Autodesk Fusion 360 part; units mm, degrees
(part 2 of 2)
sketch "Sketch30" plane through (0, 0, 0) normal (0, -1, 0) x (1, 0, 0)
  line L0 (40, 0) -> (71.5, 0)
  line L1 (71.5, 0) -> (71.5, 10)
  line L2 (71.5, 10) -> (40, 10)
  line L3 (40, 10) -> (40, 0)
  line L4 (40, 10) -> (42, 10)
  line L5 (42, 10) -> (40, 0)
  line L6 (40, 0) -> (40, 10)
  line L7 (71.5, 10) -> (69.5, 10)
  line L8 (69.5, 10) -> (71.5, 0)
  line L9 (71.5, 0) -> (71.5, 10)
  dimension "d261" = 2
  constraint coincident L2.end L3.start
  constraint coincident L2 L4.end
  constraint coincident L0.start L3.end
  constraint coincident L1.end L2.start
  constraint perpendicular L1 L7
  constraint coincident L0.end L1.start
  measures "d261" distance of L1.end L7.end
sketch "Sketch31" plane through (71.5, 0, 0) normal (1, 0, 0) x (0, 0, -1)
  line L0 (0, 0) -> (0, 18)
  line L1 (0, 18) -> (-10, 18)
  line L2 (-10, 18) -> (-10, 0)
  line L3 (-10, 0) -> (0, 0)
  line L4 (-10, 0) -> (-10, 2)
  line L5 (-10, 2) -> (0, 0)
  line L6 (0, 0) -> (-10, 0)
  line L7 (-10, 18) -> (-10, 16)
  line L8 (-10, 16) -> (0, 18)
  line L9 (0, 18) -> (-10, 18)
  constraint coincident L2.end L3.start
  constraint coincident L2 L4.end
  constraint coincident L0.start L3.end
  constraint coincident L1.end L2.start
  constraint coincident L2 L7.end
  constraint coincident L0.end L1.start
extrude "Extrude32" cut sketch "Sketch31" against normal blind 40 contours L2 L3 L4 L5 L6 | L1 L2 L7 L8 L9 bodies 8
extrude "Extrude33" cut sketch "Sketch30" against normal blind 27 contours L2 L3 L4 L5 L6 | L1 L2 L7 L8 L9 bodies 8
shell "Shell9" thickness 1 removed faces 1 at (50.5, 12, 0) on bodies 8
sketch "Sketch32" plane through (0, 0, 9) normal (0, 0, -1) x (-1, 0, 0)
  line L0 (-68.6802, 15.1802) -> (-68.6802, 2.8198)
  line L1 (-68.6802, 2.8198) -> (-42.8198, 2.8198)
  line L2 (-42.8198, 2.8198) -> (-42.8198, 15.1802)
  line L3 (-42.8198, 15.1802) -> (-68.6802, 15.1802)
  line L4 (-56.3, 7) -> (-55.2, 7)
  line L5 (-55.2, 7) -> (-55.2, 11)
  line L6 (-55.2, 11) -> (-56.3, 11)
  line L7 (-56.3, 11) -> (-56.3, 7)
  line L8 (-53.75, 8.375) -> (-57.75, 8.375)
  line L9 (-57.75, 8.375) -> (-57.75, 9.625)
  line L10 (-57.75, 9.625) -> (-53.75, 9.625)
  line L11 (-53.75, 9.625) -> (-53.75, 8.375)
  line L12 (-57.3, 6) -> (-54.2, 6)
  line L13 (-54.2, 6) -> (-54.2, 12)
  line L14 (-54.2, 12) -> (-57.3, 12)
  line L15 (-57.3, 12) -> (-57.3, 6)
  line L16 (-58.75, 10.625) -> (-52.75, 10.625)
  line L17 (-52.75, 10.625) -> (-52.75, 7.375)
  line L18 (-52.75, 7.375) -> (-58.75, 7.375)
  line L19 (-58.75, 7.375) -> (-58.75, 10.625)
  dimension "d275" = 3.1
  dimension "d276" = 6
  dimension "d279" = 6
  dimension "d280" = 3.25
  constraint horizontal L4
  constraint vertical L5
  constraint horizontal L6
  constraint vertical L7
  constraint horizontal L8
  constraint vertical L9
  constraint horizontal L10
  constraint vertical L11
  constraint horizontal L12
  constraint vertical L13
  constraint horizontal L14
  constraint vertical L15
  constraint horizontal L16
  constraint vertical L17
  constraint horizontal L18
  constraint vertical L19
  measures "d275" distance of L12.start L12.end
  measures "d276" distance of L12.start L14.end
  measures "d279" distance of L16.start L16.end
  measures "d280" distance of L16.start L18.end
extrude "Extrude34" add sketch "Sketch32" along normal blind 9 contours L4 L5 L7 L12 L13 L15 L18 | L7 L8 L15 L18 | L5 L8 L13 L18 | L8 L9 L10 L15 L16 L18 L19 | L8 L10 L11 L13 L16 L17 L18 | L7 L10 L15 L16 | L5 L10 L13 L16 | L5 L6 L7 L13 L14 L15 L16 bodies 8
fillet "Fillet9" radius 1 8 edges at (55.75, 16, 10) (41, 17, 5) (42, 9, 10) (41, 1, 5) (55.75, 2, 10) (70.5, 17, 5) (69.5, 9, 10) (70.5, 1, 5) on bodies 8
move_body "Move13" bodies 8 to x (1, 0, 0) y (0, 1, 0) z (0, 0, 1) at (-55.7506, -8.335, 12.2427)
move_body "Move14" bodies 1 to x (1, 0, 0) y (0, 1, 0) z (0, 0, 1) at (70, 0, 0)
move_body "Move15" bodies 2 to x (1, 0, 0) y (0, 1, 0) z (0, 0, 1) at (-80, 0, 0)
move_body "Move16" bodies 3 to x (1, 0, 0) y (0, 1, 0) z (0, 0, 1) at (100, 0, 0)
move_body "Move17" bodies 4 to x (1, 0, 0) y (0, 1, 0) z (0, 0, 1) at (140, 0, 0)
move_body "Move18" bodies 5 to x (1, 0, 0) y (0, 1, 0) z (0, 0, 1) at (180, 0, 0)
move_body "Move19" bodies 6 to x (1, 0, 0) y (0, 1, 0) z (0, 0, 1) at (220, 0, 0)
move_body "Move20" bodies 7 to x (1, 0, 0) y (0, 1, 0) z (0, 0, 1) at (270, 0, 0)
move_body "Move21" bodies 8 to x (1, 0, 0) y (0, 1, 0) z (0, 0, 1) at (40, 0, 0)
move_body "Move22" bodies 2 to x (1, 0, 0) y (0, 1, 0) z (0, 0, 1) at (40, 0, 0)
sketch "Sketch33" plane through (0, 0, 0) normal (0, 0, 1) x (1, 0, 0)
  line L0 (-280, 0) -> (-167.5, 0)
  line L1 (-167.5, 0) -> (-167.5, 18)
  line L2 (-167.5, 18) -> (-280, 18)
  line L3 (-280, 18) -> (-280, 0)
  dimension "d285" = 112.5
  dimension "d286" = 18
  constraint horizontal L0
  constraint vertical L1
  constraint horizontal L2
  constraint vertical L3
  measures "d285" distance of L0.start L0.end
  measures "d286" distance of L0.start L2.end
extrude "Extrude35" add sketch "Sketch33" along normal blind 10 separate body makes body 9
sketch "Sketch34" plane through (0, 0, 0) normal (0, -1, 0) x (1, 0, 0)
  line L0 (-280, 0) -> (-167.5, 0)
  line L1 (-167.5, 0) -> (-167.5, 10)
  line L2 (-167.5, 10) -> (-280, 10)
  line L3 (-280, 10) -> (-280, 0)
  line L4 (-167.5, 10) -> (-169.5, 10)
  line L5 (-169.5, 10) -> (-167.5, 0)
  line L6 (-167.5, 0) -> (-167.5, 10)
  line L7 (-280, 10) -> (-278, 10)
  line L8 (-278, 10) -> (-280, 0)
  line L9 (-280, 0) -> (-280, 10)
  dimension "d289" = 2
  dimension "d290" = 2
  constraint coincident L1.end L2.start
  constraint perpendicular L1 L4
  constraint coincident L0.end L1.start
  constraint coincident L2.end L3.start
  constraint perpendicular L3 L7
  constraint coincident L0.start L3.end
  measures "d289" distance of L1.end L4.end
  measures "d290" distance of L2.end L7.end
sketch "Sketch35" plane through (-280, 0, 0) normal (-1, 0, 0) x (0, 0, 1)
  line L0 (0, 18) -> (0, 0)
  line L1 (0, 0) -> (10, 0)
  line L2 (10, 0) -> (10, 18)
  line L3 (10, 18) -> (0, 18)
  line L4 (10, 18) -> (10, 16)
  line L5 (10, 16) -> (0, 18)
  line L6 (0, 18) -> (10, 18)
  line L7 (10, 0) -> (10, 2)
  line L8 (10, 2) -> (0, 0)
  line L9 (0, 0) -> (10, 0)
  dimension "d291" = 2
  dimension "d292" = 2
  constraint coincident L2.end L3.start
  constraint perpendicular L3 L4
  constraint coincident L0.start L3.end
  constraint coincident L1.end L2.start
  constraint perpendicular L1 L7
  constraint coincident L0.end L1.start
  measures "d291" distance of L2.end L4.end
  measures "d292" distance of L1.end L7.end
extrude "Extrude36" cut sketch "Sketch35" against normal blind 120 contours L2 L3 L4 L5 L6 | L1 L2 L7 L8 L9 bodies 9
extrude "Extrude37" cut sketch "Sketch34" against normal blind 35 contours L2 L3 L7 L8 L9 | L1 L2 L4 L5 L6 bodies 9
shell "Shell10" thickness 1 removed faces 1 at (-242.5, 6, 0) on bodies 9
sketch "Sketch36" plane through (0, 0, 9) normal (0, 0, -1) x (-1, 0, 0)
  line L0 (277.1802, 2.8198) -> (277.1802, 15.1802)
  line L1 (277.1802, 15.1802) -> (170.3198, 15.1802)
  line L2 (170.3198, 15.1802) -> (170.3198, 2.8198)
  line L3 (170.3198, 2.8198) -> (277.1802, 2.8198)
  line L4 (224.3, 7) -> (223.2, 7)
  line L5 (223.2, 7) -> (223.2, 11)
  line L6 (223.2, 11) -> (224.3, 11)
  line L7 (224.3, 11) -> (224.3, 7)
  line L8 (225.75, 9.625) -> (221.75, 9.625)
  line L9 (221.75, 9.625) -> (221.75, 8.375)
  line L10 (221.75, 8.375) -> (225.75, 8.375)
  line L11 (225.75, 8.375) -> (225.75, 9.625)
  line L12 (222.2, 6) -> (225.3, 6)
  line L13 (225.3, 6) -> (225.3, 12)
  line L14 (225.3, 12) -> (222.2, 12)
  line L15 (222.2, 12) -> (222.2, 6)
  line L16 (220.75, 10.625) -> (226.75, 10.625)
  line L17 (226.75, 10.625) -> (226.75, 7.375)
  line L18 (226.75, 7.375) -> (220.75, 7.375)
  line L19 (220.75, 7.375) -> (220.75, 10.625)
  line L20 (176.469, 7.375) -> (170.469, 7.375)
  line L21 (170.469, 7.375) -> (170.469, 10.625)
  line L22 (170.469, 10.625) -> (176.469, 10.625)
  line L23 (176.469, 10.625) -> (176.469, 7.375)
  line L24 (171.469, 8.375) -> (175.469, 8.375)
  line L25 (175.469, 8.375) -> (175.469, 9.625)
  line L26 (171.469, 9.625) -> (171.469, 8.375)
  line L27 (175.469, 9.625) -> (171.469, 9.625)
  line L28 (174.019, 11) -> (174.019, 7)
  line L29 (174.019, 7) -> (172.919, 7)
  line L30 (172.919, 11) -> (174.019, 11)
  line L31 (172.919, 7) -> (172.919, 11)
  line L32 (171.919, 6) -> (175.019, 6)
  line L33 (175.019, 6) -> (175.019, 12)
  line L34 (171.919, 12) -> (171.919, 6)
  line L35 (175.019, 12) -> (171.919, 12)
  line L36 (277.031, 7.375) -> (271.031, 7.375)
  line L37 (271.031, 7.375) -> (271.031, 10.625)
  line L38 (271.031, 10.625) -> (277.031, 10.625)
  line L39 (277.031, 10.625) -> (277.031, 7.375)
  line L40 (272.031, 8.375) -> (276.031, 8.375)
  line L41 (276.031, 8.375) -> (276.031, 9.625)
  line L42 (272.031, 9.625) -> (272.031, 8.375)
  line L43 (276.031, 9.625) -> (272.031, 9.625)
  line L44 (274.581, 11) -> (274.581, 7)
  line L45 (274.581, 7) -> (273.481, 7)
  line L46 (273.481, 11) -> (274.581, 11)
  line L47 (273.481, 7) -> (273.481, 11)
  line L48 (272.481, 6) -> (275.581, 6)
  line L49 (275.581, 6) -> (275.581, 12)
  line L50 (272.481, 12) -> (272.481, 6)
  line L51 (275.581, 12) -> (272.481, 12)
  dimension "d310" = 3.1
  dimension "d311" = 6
  dimension "d314" = 6
  dimension "d315" = 3.25
  dimension "d316" = 3.1
  dimension "d317" = 6
  dimension "d318" = 6
  dimension "d319" = 3.25
  dimension "d320" = 3.1
  dimension "d321" = 6
  dimension "d322" = 6
  dimension "d323" = 3.25
  constraint horizontal L4
  constraint vertical L5
  constraint horizontal L6
  constraint vertical L7
  constraint horizontal L8
  constraint vertical L9
  constraint horizontal L10
  constraint vertical L11
  constraint horizontal L12
  constraint vertical L13
  constraint horizontal L14
  constraint vertical L15
  constraint horizontal L16
  constraint vertical L17
  constraint horizontal L18
  constraint vertical L19
  constraint horizontal L29
  constraint vertical L31
  constraint horizontal L30
  constraint vertical L28
  constraint horizontal L27
  constraint vertical L26
  constraint horizontal L24
  constraint vertical L25
  constraint horizontal L32
  constraint vertical L33
  constraint horizontal L35
  constraint vertical L34
  constraint horizontal L22
  constraint vertical L23
  constraint horizontal L20
  constraint vertical L21
  constraint horizontal L45
  constraint vertical L47
  constraint horizontal L46
  constraint vertical L44
  constraint horizontal L43
  constraint vertical L42
  constraint horizontal L40
  constraint vertical L41
  constraint horizontal L48
  constraint vertical L49
  constraint horizontal L51
  constraint vertical L50
  constraint horizontal L38
  constraint vertical L39
  constraint horizontal L36
  constraint vertical L37
  measures "d310" distance of L12.start L12.end
  measures "d311" distance of L12.start L14.end
  measures "d314" distance of L16.start L16.end
  measures "d315" distance of L16.start L18.end
  measures "d316" distance of L32.start L32.end
  measures "d317" distance of L32.start L34.start
  measures "d318" distance of L21.end L22.end
  measures "d319" distance of L20.end L21.end
  measures "d320" distance of L48.start L48.end
  measures "d321" distance of L48.start L50.start
  measures "d322" distance of L37.end L38.end
  measures "d323" distance of L36.end L37.end
extrude "Extrude38" add sketch "Sketch36" along normal blind 9 contours L4 L5 L7 L12 L13 L15 L18 | L7 L10 L13 L18 | L5 L10 L15 L18 | L8 L10 L11 L13 L16 L17 L18 | L8 L9 L10 L15 L16 L18 L19 | L7 L8 L13 L16 | L5 L8 L15 L16 | L5 L6 L7 L13 L14 L15 L16 | L20 L22 L23 L24 L25 L27 L33 | L20 L28 L29 L31 L32 L33 L34 | L20 L24 L28 L33 | L22 L27 L28 L33 | L22 L28 L30 L31 L33 L34 L35 | L20 L24 L31 L34 | L20 L21 L22 L24 L26 L27 L34 | L22 L27 L31 L34 | L36 L38 L39 L40 L41 L43 L49 | L36 L44 L45 L47 L48 L49 L50 | L36 L40 L44 L49 | L38 L43 L44 L49 | L38 L44 L46 L47 L49 L50 L51 | L36 L40 L47 L50 | L36 L37 L38 L40 L42 L43 L50 | L38 L43 L47 L50 bodies 9
fillet "Fillet10" radius 1 8 edges at (-223.75, 16, 10) (-279, 17, 5) (-278, 9, 10) (-279, 1, 5) (-223.75, 2, 10) (-168.5, 17, 5) (-169.5, 9, 10) (-168.5, 1, 5) on bodies 9
move_body "Move23" bodies 9 to x (1, 0, 0) y (0, 1, 0) z (0, 0, 1) at (78.9681, -8.3243, 12.2055)
move_body "Move24" bodies 9 to x (1, 0, 0) y (0, 1, 0) z (0, 0, 1) at (100, 0, 0)
hidden bodies 2
equation "d31 = 18 mm + 18 mm + 18 mm + 18 mm + 18 mm + 18 mm"
equation "d70 = 18 mm + 4.5 mm"
equation "d100 = 18 mm + 18 mm"
equation "d150 = 18 mm + 9 mm"
equation "d174 = 18 mm + 18 mm + 4.5 mm"
equation "d212 = 18 mm + 18 mm + 9 mm + 4.5 mm"
equation "d257 = 18 mm + 9 mm + 4.5 mm"
equation "d285 = 18 mm + 18 mm + 18 mm + 18 mm + 18 mm + 18 mm + 4.5 mm"
